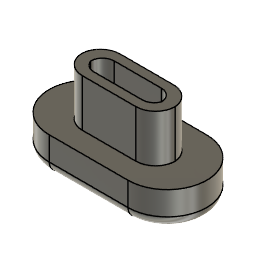
pmsa003i_air_intake_seperator (Autodesk Fusion 360 design; units mm, degrees)
part number: 2026-04-25-15-49-09-861
Autodesk Fusion 360 part; units mm, degrees
sketch "Sketch1" plane through (0, 0, 0) normal (0, 0, 1) x (1, 0, 0)
  line L0 (5.9, -2.4) -> (-5.9, -2.4)
  line L1 (-5.9, -2.4) -> (-5.9, 2.4)
  line L2 (-5.9, 2.4) -> (5.9, 2.4)
  line L3 (5.9, 2.4) -> (5.9, -2.4)
  line L4 (5.9, -2.4) -> (-5.9, 2.4) construction
  line L5 (-5.9, -2.4) -> (5.9, 2.4) construction
  line L6 (4.5, 1.25) -> (-4.5, 1.25)
  line L7 (-4.5, 1.25) -> (-4.5, -1.25)
  line L8 (-4.5, -1.25) -> (4.5, -1.25)
  line L9 (4.5, -1.25) -> (4.5, 1.25)
  line L10 (4.5, 1.25) -> (-4.5, -1.25) construction
  line L11 (-4.5, 1.25) -> (4.5, -1.25) construction
  line L12 (10, -5) -> (-10, -5)
  line L13 (-10, -5) -> (-10, 5)
  line L14 (-10, 5) -> (10, 5)
  line L15 (10, 5) -> (10, -5)
  line L16 (10, -5) -> (-10, 5) construction
  line L17 (-10, -5) -> (10, 5) construction
  dimension "d1" = 4.8
  dimension "d2" = 11.8
  dimension "d3" = 9
  dimension "d4" = 2.5
  dimension "d5" = 20
  dimension "d6" = 10
  constraint horizontal L0
  constraint perpendicular L0 L1
  constraint parallel L0 L2
  constraint parallel L1 L3
  constraint coincident L4 origin
  constraint coincident L5 origin
  constraint horizontal L6
  constraint perpendicular L6 L7
  constraint parallel L6 L8
  constraint parallel L7 L9
  constraint coincident L10 origin
  constraint coincident L11 origin
  constraint horizontal L12
  constraint perpendicular L12 L13
  constraint parallel L12 L14
  constraint parallel L13 L15
  constraint coincident L16 origin
  constraint coincident L17 origin
  measures "d1" distance of L0.end L1.end
  measures "d2" distance of L1 L3
  measures "d3" distance of L7.end L8.end
  measures "d4" distance of L6.end L7.end
  measures "d5" distance of L13.end L14.end
  measures "d6" distance of L12.end L13.end
extrude "Extrude1" add sketch "Sketch1" along normal blind 4.5 contours L12 L13 L14 L15
extrude "Extrude2" add sketch "Sketch1" along normal blind 10.5 contours L0 L1 L2 L3
fillet "Fillet1" radius 1.5 4 edges at (4.5, 1.25, 5.25) (-4.5, 1.25, 5.25) (-4.5, -1.25, 5.25) (4.5, -1.25, 5.25)
fillet "Fillet2" radius 2.5 4 edges at (-5.9, -2.4, 7.5) (-5.9, 2.4, 7.5) (5.9, -2.4, 7.5) (5.9, 2.4, 7.5)
fillet "Fillet3" radius 5 4 edges at (-10, 5, 2.25) (-10, -5, 2.25) (10, -5, 2.25) (10, 5, 2.25)
fillet "Fillet4" radius 1.5 4 edges at (10, 0, 0) (0, -5, 0) (-10, 0, 0) (0, 5, 0)
extrude "Extrude3" cut sketch "Sketch1" along normal blind 2.5 contours L0 L1 L2 L3 | L6 L7 L8 L9
chamfer "Chamfer1" distance 1 angle 45 6 edges at (4.0607, 0.8107, 2.5) (-4.0607, 0.8107, 2.5) (0, 1.25, 2.5) (-3.9518, -0.9747, 2.5) (3.9518, -0.9747, 2.5) (0, -1.25, 2.5)
fillet "Fillet5" radius 2.5 4 edges at (5.9, 2.4, 1.25) (5.9, -2.4, 1.25) (-5.9, -2.4, 1.25) (-5.9, 2.4, 1.25)
fillet "Fillet6" radius 0.25 6 edges at (5.0999, -1.7331, 2.5) (0.004, -2.4, 2.5) (-5.1678, -1.6678, 2.5) (-5.0999, 1.7331, 2.5) (-0.004, 2.4, 2.5) (5.1678, 1.6678, 2.5)
fillet "Fillet7" radius 0.5 6 edges at (-5.0999, 1.7331, 0) (-0.004, 2.4, 0) (5.1678, 1.6678, 0) (-5.1678, -1.6678, 0) (0.004, -2.4, 0) (5.0999, -1.7331, 0)
